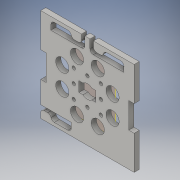
# Autodesk Inventor part: BottomRotated
Saved by Autodesk Inventor 2016 SP1 (Build 200210100, 210)
## iProperties
Created: 2015-06-30
Part Number: BottomRotated
Material: Generic
Document SubType Name: Modeling
Designer: Rodrigo
Density: 1 g/cm^3
Appearance: Default
Author: Rodrigo
Autodesk Inventor part; units mm, degrees
ref_plane "YZ Plane" through (0, 0, 0) normal (1, 0, 0) x (0, 1, 0)
ref_plane "XZ Plane" through (0, 0, 0) normal (0, 1, 0) x (-1, 0, 0)
ref_plane "XY Plane" through (0, 0, 0) normal (0, 0, 1) x (1, 0, 0)
ref_plane "Work Plane1" through (0, 0, 0) normal (0, 0, 1) x (1, 0, 0)
sketch "Sketch1" plane through (0, 0, 0) normal (0, 0, 1) x (1, 0, 0)
  circle A0 centre (6.5, 20.75) radius 1
  circle A1 centre (6.5, 4.75) radius 1
  circle A2 centre (22.5, 20.75) radius 1
  circle A3 centre (22.5, 4.75) radius 1
  line L0 (-13, -14.75) -> (42, -14.75)
  line L1 (42, -14.75) -> (42, 40.25)
  line L2 (42, 40.25) -> (-13, 40.25)
  line L3 (-13, 40.25) -> (-13, -14.75)
  line L4 (-13, -14.75) -> (42, 40.25) construction
  line L5 (42, -14.75) -> (-13, 40.25) construction
  circle A4 centre (22.5, 12.75) radius 1 projected
  circle A5 centre (14.5, 20.75) radius 1 projected
  circle A6 centre (14.5, 4.75) radius 1 projected
  circle A7 centre (6.5, 12.75) radius 1 projected
  line L6 (19.5, 15.75) -> (19.5, 9.75)
  line L7 (17.1458, 15.75) -> (19.5, 15.75)
  arc A8 (17.1458, 15.75) -> (11.8542, 15.75) centre (14.5, 12.75) ccw
  line L8 (9.5, 15.75) -> (11.8542, 15.75)
  line L9 (9.5, 9.75) -> (9.5, 15.75)
  line L10 (11.8542, 9.75) -> (9.5, 9.75)
  arc A9 (11.8542, 9.75) -> (17.1458, 9.75) centre (14.5, 12.75) ccw
  line L11 (19.5, 9.75) -> (17.1458, 9.75)
  point P0 (0, 0)
  dimension "d0" = 55
  dimension "d1" = 55
  dimension "d95" = 2
  dimension "d96" = 2
  dimension "d97" = 2
  dimension "d98" = 2
  constraints: 24 end point, 6 centre point, 4 point on circle, 2 midpoint, 2 parallel, 1 horizontal, 1 perpendicular
  measures "d0" distance of L2.end L1.end
  measures "d1" distance of L1.end L0.end
  measures "d95" diameter of A0
  measures "d96" diameter of A2
  measures "d97" diameter of A3
  measures "d98" diameter of A1
extrude "Extrusion3" add sketch "Sketch1" along normal blind 3
sketch "Sketch4" plane through (0, 0, 3) normal (0, 0, 1) x (1, 0, 0)
  line L0 (14.5, 40.25) -> (14.5, 12.75) construction
  line L1 (-13, -14.75) -> (42, -14.75) construction
  line L2 (-13, 12.75) -> (14.5, 12.75) construction
  line L3 (5, 38.25) -> (-7, 38.25)
  line L4 (-7, 38.25) -> (-7, 33.25)
  line L5 (-7, 33.25) -> (13, 33.25)
  line L6 (13, 40.25) -> (13, 33.25)
  line L7 (-7, -12.75) -> (5, -12.75)
  line L8 (5, -12.75) -> (5, -7.75)
  line L9 (5, -7.75) -> (-13, -7.75)
  line L10 (-13, -14.75) -> (-13, -7.75)
  line L11 (-13, -14.75) -> (5.3284, -14.75)
  line L12 (14.5, 12.75) -> (20.6229, 27.5321)
  line L13 (14.5, 12.75) -> (30.5, 12.75) construction
  circle A0 centre (20.6229, 27.5321) radius 3.895
  circle A1 centre (8.3771, 27.5321) radius 3.895
  circle A2 centre (-0.2821, 18.8729) radius 3.895
  circle A3 centre (-0.2821, 6.6271) radius 3.895
  circle A4 centre (8.3771, -2.0321) radius 3.895
  circle A5 centre (20.6229, -2.0321) radius 3.895
  circle A6 centre (29.2821, 6.6271) radius 3.895
  circle A7 centre (29.2821, 18.8729) radius 3.895
  line L14 (-7, -12.75) -> (-7, -9.75)
  line L15 (-7, -9.75) -> (-13, -9.75)
  line L16 (-13, 40.25) -> (-13, -14.75) projected
  line L17 (-13, -7.75) -> (-13, -9.75)
  line L18 (-13, 40.25) -> (-13, -14.75) projected
  line L19 (5, 38.25) -> (5, 35.25)
  line L20 (5, 35.25) -> (11, 35.25)
  line L21 (11, 35.25) -> (11, 40.25)
  line L22 (42, 40.25) -> (-13, 40.25) projected
  line L23 (42, 40.25) -> (-13, 40.25) projected
  line L24 (11, 40.25) -> (13, 40.25)
  line L25 (24, 38.25) -> (36, 38.25)
  line L26 (36, 38.25) -> (36, 33.25)
  line L27 (36, 33.25) -> (16, 33.25)
  line L28 (16, 40.25) -> (16, 33.25)
  line L29 (24, 38.25) -> (24, 35.25)
  line L30 (24, 35.25) -> (18, 35.25)
  line L31 (18, 35.25) -> (18, 40.25)
  line L32 (18, 40.25) -> (16, 40.25)
  point P0 (0, 0)
  dimension "d99" = 16
  dimension "d100" = 67.5
  dimension "d101" = 7.79
  dimension "d104" = 360
  dimension "d106" = 2
  dimension "d107" = 5
  dimension "d108" = 2
  dimension "d109" = 12
  dimension "d110" = 18
  dimension "d111" = 6
  dimension "d112" = 20
  dimension "d113" = 12
  dimension "d114" = 6
  dimension "d115" = 5
  dimension "d117" = 2
  dimension "d118" = 2
  constraints: 58 end point, 8 centre point, 8 symmetric about line, 5 vertical, 4 perpendicular, 3 collinear, 3 horizontal, 2 point on line, 1 coincident, 1 equal length, 17 other
  measures "d99" distance of L0.end L12.end
  measures "d100" angle of L13 L12
  measures "d101" diameter of A0
  measures "d106" distance between parallel lines of L1 L7
  measures "d107" distance between parallel lines of L1 L15
  measures "d108" distance between parallel lines of L15 L9
  measures "d109" distance of L7.start L7.end
  measures "d110" distance of L8.end L9.end
  measures "d111" distance between parallel lines of L16 L4
  measures "d112" distance between parallel lines of L6 L4
  measures "d113" distance of L3.start L3.end
  measures "d114" distance of L19.end L20.end
  measures "d115" distance of L20.end L21.end
  measures "d117" distance between parallel lines of L22 L3
  measures "d118" distance between parallel lines of L20 L5
extrude "Extrusion2" cut sketch "Sketch4" against normal through all
fillet "Fillet3" radius 2 14 edges at (-7, 38.25, 1.5) (5, 38.25, 1.5) (13, 33.25, 1.5) (5, -12.75, 1.5) (-7, -12.75, 1.5) (-7, -9.75, 1.5) (-13, -9.75, 1.5) (5, 35.25, 1.5) (11, 35.25, 1.5) (18, 35.25, 1.5) (24, 35.25, 1.5) (24, 38.25, 1.5) (36, 38.25, 1.5) (16, 33.25, 1.5)
sketch "Sketch6" plane through (0, 0, 3) normal (0, 0, 1) x (1, 0, 0)
  line L0 (38.85, 20.3) -> (42, 20.3)
  line L1 (42, 20.3) -> (42, 5.2)
  line L2 (42, 5.2) -> (38.85, 5.2)
  line L3 (38.85, 5.2) -> (38.85, 20.3)
  line L4 (42, -14.75) -> (42, 40.25) projected
  line L5 (42, 40.25) -> (-13, 40.25) construction
  line L6 (14.5, 40.25) -> (14.5, -14.75) construction
  line L7 (-13, -14.75) -> (42, -14.75) construction
  line L8 (-9.85, 20.3) -> (-13, 20.3)
  line L9 (-13, 5.2) -> (-9.85, 5.2)
  line L10 (-9.85, 5.2) -> (-9.85, 20.3)
  line L11 (-13, 12.75) -> (42, 12.75) construction
  line L12 (-13, 20.3) -> (-13, 5.2)
  line L13 (-13, 40.25) -> (-13, -14.75) projected
  point P0 (0, 0)
  point P1 (42, 12.75)
  point P2 (18.0284, 40.25)
  point P3 (13, 40.25)
  point P4 (5.3284, -14.75)
  point P5 (-13, 12.75)
  point P6 (-13, -7.75)
  dimension "d91" = 3.15
  dimension "d92" = 15.1
  constraints: 20 end point, 8 symmetric about line, 4 midpoint, 2 horizontal, 2 parallel, 1 coincident, 1 collinear, 1 perpendicular, 1 point on line, 1 vertical
  measures "d91" distance of L1.end L2.end
  measures "d92" distance of L0.end L1.end
extrude "Extrusion4" cut sketch "Sketch6" against normal through all
equation "\"d38\" = d24"
equation "\"d24\" = 7.79"
body "Solid1"
body "Solid2"
